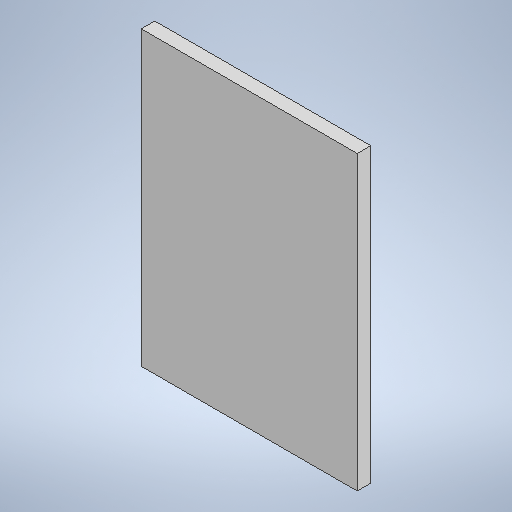
# Autodesk Inventor part: carcasa_piezaLateral_ruedas
Saved by Autodesk Inventor 2025.3 (Build 293356030, 356C)
## iProperties
Created: 2025-09-08
Part Number: carcasa_piezaLateral_ruedas
Material: Generic
Document SubType Name: Modeling
Designer: brene
Density: 1 g/cm^3
Appearance: Default
Author: brene
Autodesk Inventor part; units mm, degrees
ref_plane "YZ Plane" through (0, 0, 0) normal (1, 0, 0) x (0, 1, 0)
ref_plane "XZ Plane" through (0, 0, 0) normal (0, 1, 0) x (-1, 0, 0)
ref_plane "XY Plane" through (0, 0, 0) normal (0, 0, 1) x (1, 0, 0)
sketch "Sketch1" plane through (0, 0, 0) normal (0, 0, 1) x (1, 0, 0)
  line L0 (0, 0) -> (48.026, 0)
  line L1 (48.026, 0) -> (48.026, 65)
  line L2 (48.026, 65) -> (0, 65)
  line L3 (0, 65) -> (0, 0)
  dimension "d0" = 48.026
  dimension "d1" = 65
  dimension "d2" = 48.026
  constraints: 8 end point, 2 perpendicular, 1 horizontal
  measures "d0" distance of L0.start L0.end
  measures "d1" distance of L0.end L1.end
  measures "d2" distance of L1.end L2.end
extrude "Extrusion1" add sketch "Sketch1" along normal blind 3
sketch "Sketch2" plane through (0, 0, 0) normal (0, -1, 0) x (1, 0, 0)
  point P0 (0, 0)
body "Solid1"
